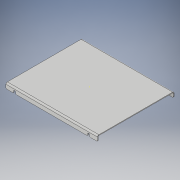
# Autodesk Inventor part: Boden
Saved by Autodesk Inventor 2018 (Build 220112000, 112)
## iProperties
Created: 2017-11-12
Part Number: Boden
Material: Generisch
Document SubType Name: Blech
Density: 1 g/cm^3
Sheet Metal Rule: Standard_mm
Appearance: Vorgabe
Autodesk Inventor part; units mm, degrees
ref_plane "YZ Plane" through (0, 0, 0) normal (1, 0, 0) x (0, 1, 0)
ref_plane "XZ Plane" through (0, 0, 0) normal (0, 1, 0) x (-1, 0, 0)
ref_plane "XY Plane" through (0, 0, 0) normal (0, 0, 1) x (1, 0, 0)
sketch "Skizze1" plane through (0, 0, 0) normal (0, 0, 1) x (1, 0, 0)
  line L0 (-131.4, -109.9) -> (131.4, -109.9)
  line L1 (131.4, -109.9) -> (131.4, 109.9)
  line L2 (131.4, 109.9) -> (-131.4, 109.9)
  line L3 (-131.4, 109.9) -> (-131.4, -109.9)
  line L4 (-131.4, -109.9) -> (131.4, 109.9) construction
  line L5 (131.4, -109.9) -> (-131.4, 109.9) construction
  point P0 (0, 0)
  dimension "d0" = 262.8
  dimension "d1" = 219.8
  measures "d0" distance of L2.end L1.end
  measures "d1" distance of L1.end L0.end
extrude "Grobblech1" add sketch "Skizze1" along normal blind 2
sketch "Skizze4" plane through (-131.4, -107.9, 2) normal (0, -1, 0) x (1, 0, 0)
  line L0 (262.8, 0) -> (0, 0)
  line L1 (0, 0) -> (0, -15)
  line L2 (0, -15) -> (262.8, -15)
  line L3 (262.8, -15) -> (262.8, 0)
  constraints: 6 end point, 1 horizontal, 1 perpendicular, 1 vertical
edge flange "Lasche3" height 15 angle 90 thickness 2 bend radius 2 thickness toward (0, -1, 0) relief straight relief width 2 relief depth 1 corner gap 2 corner form 0 edges at (0, -109.9, 0) (0, 109.9, 0) wall of the first edge with corners at (131.4, -107.9, 2) (-131.4, -107.9, 2) (-131.4, -107.9, -13) (131.4, -107.9, -13)
bend "Biegung3"
corner "Ecke3"
sketch "Skizze5" plane through (-131.4, -109.9, -13) normal (0, -1, 0) x (1, 0, 0)
  line L0 (131.4, -3.4971) -> (131.4, 18.0828) construction
  circle A0 centre (237.8, 5) radius 3.15
  line L1 (262.8, 11) -> (262.8, 0) construction
  line L2 (262.8, 0) -> (0, 0) construction
  line L3 (0, 0) -> (262.8, 0) construction
  line L4 (234.65, 5) -> (234.65, 2)
  line L5 (240.95, 5) -> (240.95, 2)
  line L6 (232.65, 0) -> (131.4, 0)
  arc A1 (232.65, 0) -> (234.65, 2) centre (232.65, 2) ccw
  line L7 (242.95, 0) -> (262.8, 0)
  arc A2 (240.95, 2) -> (242.95, 0) centre (242.95, 2) ccw
  circle A3 centre (25, 5) radius 3.15
  line L8 (0, 0) -> (262.8, 0) construction
  line L9 (262.8, 0) -> (0, 0) construction
  line L10 (28.15, 5) -> (28.15, 2)
  line L11 (21.85, 5) -> (21.85, 2)
  line L12 (30.15, 0) -> (131.4, 0)
  arc A4 (28.15, 2) -> (30.15, 0) centre (30.15, 2) ccw
  line L13 (19.85, 0) -> (0, 0)
  arc A5 (19.85, 0) -> (21.85, 2) centre (19.85, 2) ccw
  line L14 (19.85, 0) -> (30.15, 0)
  line L15 (232.65, 0) -> (242.95, 0)
  point P0 (131.4, 13)
  point P1 (234.65, 0)
  point P2 (240.95, 0)
  point P3 (28.15, 0)
  point P4 (21.85, 0)
  dimension "d33" = 6.3
  dimension "d34" = 25
  dimension "d35" = 5
  dimension "d36" = 2
  dimension "d37" = 2
  constraints: 24 end point, 13 symmetric about line, 12 point on circle, 12 point on line, 8 tangent, 6 centre point, 3 collinear, 2 perpendicular, 1 midpoint, 3 other
  measures "d33" diameter of A0
  measures "d34" distance from line of L1 A0.centre
  measures "d35" distance from line of L2 A0.centre
  measures "d36" radius of A1
  measures "d37" radius of A2
extrude "Extrusion1" cut sketch "Skizze5" against normal through all
fillet "Rundung1" radius 2 4 edges at (131.4, -108.9, -13) (131.4, 108.9, -13) (-131.4, -108.9, -13) (-131.4, 108.9, -13)
equation "\"d2\" = Stärke"
equation "\"d23\" = BreiteBiegungsfreistellung"
equation "\"d24\" = TiefeBiegungsfreistellung"
equation "\"d25\" = MinimalRest"
equation "\"d26\" = Übergangsradius"
equation "\"d29\" = Biegeradius"
equation "\"d30\" = GrößeEckenfreistellung"
equation "\"d31\" = Abstandsgröße"
equation "\"d32\" = JacobiRadiusGröße"
equation "\"Biegeradius\" = Stärke"
equation "\"BreiteBiegungsfreistellung\" = Stärke"
equation "\"TiefeBiegungsfreistellung\" = 0.5 * Stärke"
equation "\"GrößeEckenfreistellung\" = 4 * Stärke"
equation "\"MinimalRest\" = 2 * Stärke"
equation "\"Übergangsradius\" = Biegeradius"
equation "\"JacobiRadiusGröße\" = Biegeradius"
equation "\"Abstandsgröße\" = Stärke"
equation "\"Stärke\" = 2"
